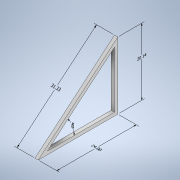
# Autodesk Inventor part: ballRampLeftSideV04-30-60
Saved by Autodesk Inventor 2020.2 (Build 242310000, 310)
## iProperties
Created: 2020-01-24
Part Number: ballRampLeftSideV04-30-60
Material: Generic
Document SubType Name: Modeling
Designer: robst
Density: 1 g/cm^3
Appearance: Default
Author: robst
Autodesk Inventor part; units mm, degrees
ref_plane "YZ Plane" through (0, 0, 0) normal (1, 0, 0) x (0, 1, 0)
ref_plane "XZ Plane" through (0, 0, 0) normal (0, 1, 0) x (-1, 0, 0)
ref_plane "XY Plane" through (0, 0, 0) normal (0, 0, 1) x (1, 0, 0)
sketch "Sketch1" plane through (0, 0, 0) normal (1, 0, 0) x (0, 1, 0)
  line L0 (0, 0) -> (0, -609.6)
  line L1 (0, -609.6) -> (511.5151, -609.6)
  line L2 (511.5151, -609.6) -> (0, 0)
  line L3 (25.4, -69.7859) -> (457.0447, -584.2)
  line L4 (457.0447, -584.2) -> (25.4, -584.2)
  line L5 (25.4, -584.2) -> (25.4, -69.7859)
  dimension "d0" = 609.6
  dimension "d1" = 40
  dimension "d2" = 25.4
  dimension "d3" = 25.4
  dimension "d4" = 25.4
  constraints: 12 end point, 2 parallel, 2 perpendicular, 1 horizontal, 1 vertical
  measures "d0" distance of L0.start L0.end
  measures "d1" angle of L2 L0
  measures "d2" distance between parallel lines of L3 L2
  measures "d3" distance between parallel lines of L5 L0
  measures "d4" distance between parallel lines of L4 L1
extrude "Extrusion1" add sketch "Sketch1" along normal mid plane 25.4
sketch "Sketch2" plane through (12.7, 0, 0) normal (1, 0, 0) x (0, 0, -1)
  line L0 (0, 0) -> (609.6, 0) projected
  line L1 (0, 0) -> (610.7413, 512.4728)
  line L2 (69.7859, 25.4) -> (584.2, 457.0447) projected
  line L3 (68.5783, 24.3867) -> (584.2, 457.0447)
  line L4 (584.2, 457.0447) -> (609.6, 478.3578)
  line L5 (584.2, 25.4) -> (69.7859, 25.4) projected
  line L6 (69.7859, 25.4) -> (39.5154, 0)
  line L7 (39.5154, 0) -> (0, 0)
  line L8 (609.6, 0) -> (609.6, 511.5151) projected
  line L9 (609.6, 511.5151) -> (609.6, 478.3578)
  point P0 (609.6, 511.5151)
  point P1 (69.7859, 25.4)
  constraints: 12 end point, 3 collinear, 2 point on line, 1 parallel
body "Solid1"
